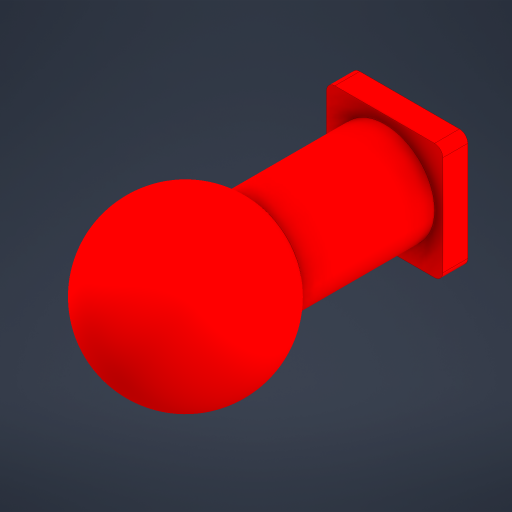
# Autodesk Inventor part: Cube Press Top
Saved by Autodesk Inventor 2023.4 (Build 274418000, 418)
## iProperties
Created: 2022-08-17
Part Number: Cube Press Top
Material: Generic
Document SubType Name: Modeling
Designer: xSibe
Density: 1 g/cm^3
Appearance: Plastic Red
Author: xSibe
Autodesk Inventor part; units mm, degrees
ref_plane "YZ Plane" through (0, 0, 0) normal (1, 0, 0) x (0, 1, 0)
ref_plane "XZ Plane" through (0, 0, 0) normal (0, 1, 0) x (-1, 0, 0)
ref_plane "XY Plane" through (0, 0, 0) normal (0, 0, 1) x (1, 0, 0)
sketch "Sketch1" plane through (0, 0, 0) normal (0, 0, 1) x (1, 0, 0)
  circle A0 centre (-21.9, -21.9) radius 1.875 projected
  circle A1 centre (21.9, 21.9) radius 1.875 projected
  circle A2 centre (21.9, -21.9) radius 1.875 projected
  circle A3 centre (-21.9, 21.9) radius 1.875 projected
  circle A4 centre (14.4, 20.8) radius 2.0734 projected
  circle A5 centre (-14.4, -20.8) radius 2.0734 projected
  circle A6 centre (14.4, -20.8) radius 2.0734 projected
  circle A7 centre (20.8, -14.4) radius 2.0734 projected
  line L0 (-17.05, 17.05) -> (-17.05, -17.05) projected
  line L1 (17.05, 17.05) -> (-17.05, 17.05) projected
  line L2 (17.05, -17.05) -> (17.05, 17.05) projected
  line L3 (-17.05, -17.05) -> (17.05, -17.05) projected
  circle A8 centre (20.8, 14.4) radius 2.0734 projected
  circle A9 centre (-14.4, 20.8) radius 2.0734 projected
  circle A10 centre (-20.8, -14.4) radius 2.0734 projected
  circle A11 centre (-20.8, 14.4) radius 2.0734 projected
  line L4 (-22.9, 24.875) -> (22.9, 24.875) projected
  arc A12 (-22.9, 24.875) -> (-24.875, 22.9) centre (-22.9, 22.9) ccw projected
  line L5 (-24.875, -22.9) -> (-24.875, 22.9) projected
  arc A13 (-24.875, -22.9) -> (-22.9, -24.875) centre (-22.9, -22.9) ccw projected
  line L6 (22.9, -24.875) -> (-22.9, -24.875) projected
  arc A14 (22.9, -24.875) -> (24.875, -22.9) centre (22.9, -22.9) ccw projected
  line L7 (24.875, 22.9) -> (24.875, -22.9) projected
  arc A15 (24.875, 22.9) -> (22.9, 24.875) centre (22.9, 22.9) ccw projected
  circle A16 centre (20.8, -14.4) radius 2.0734
  circle A17 centre (14.4, -20.8) radius 2.0734
  line L8 (-25, 25) -> (25, 25)
  line L9 (25, 25) -> (25, -25)
  line L10 (25, -25) -> (-25, -25)
  line L11 (-25, -25) -> (-25, 25)
  line L12 (-25, 25) -> (25, -25) construction
  line L13 (25, 25) -> (-25, -25) construction
  circle A18 centre (14.4, -29.2) radius 2.0734
  circle A19 centre (20.8, -35.6) radius 2.0734
  circle A20 centre (29.2, -35.6) radius 2.0734
  circle A21 centre (35.6, -29.2) radius 2.0734
  circle A22 centre (35.6, -20.8) radius 2.0734
  circle A23 centre (29.2, -14.4) radius 2.0734
  line L14 (7.5, -7.5) -> (42.5, -7.5)
  line L15 (42.5, -7.5) -> (42.5, -42.5)
  line L16 (42.5, -42.5) -> (7.5, -42.5)
  line L17 (7.5, -42.5) -> (7.5, -7.5)
  line L18 (7.5, -7.5) -> (42.5, -42.5) construction
  line L19 (42.5, -7.5) -> (7.5, -42.5) construction
  point P0 (0, 0)
  dimension "d0" = 50
  dimension "d1" = 50
  dimension "d4" = 360
  dimension "d6" = 35
  dimension "d7" = 35
  constraints: 24 end point, 8 centre point, 4 midpoint, 4 parallel, 2 coincident, 2 concentric, 2 horizontal, 2 perpendicular, 17 other
  measures "d0" distance of L9.end L10.end
  measures "d1" distance of L8.end L9.end
  measures "d6" distance of L15.end L16.end
  measures "d7" distance of L14.end L15.end
ref_plane "Work Plane1" through (-24.875, -24.875, 49.8) normal (0, 0, 1) x (1, 0, 0)
extrude "Extrusion1" add sketch "Sketch1" along normal blind 1.5 from surface at 49.8 contours A2 | L17 L14 L2 L3 | L3 L2 L14 L7 A14 L6 L17 | L6 A14 L7 L14 L9 L10 L17 | L10 L9 L14 L15 L16 L17
sketch "Sketch2" plane through (7.5, -7.5, 51.3) normal (0, 0, 1) x (1, 0, 0)
  line L0 (0, 0) -> (35, 0) projected
  line L1 (0, -35) -> (0, 0) projected
  line L2 (35, -35) -> (0, -35) projected
  line L3 (35, 0) -> (35, -35) projected
  circle A0 centre (21.7, -6.9) radius 2.0734 projected
  circle A1 centre (28.1, -21.7) radius 2.0734 projected
  circle A2 centre (13.3, -28.1) radius 2.0734 projected
  circle A3 centre (6.9, -21.7) radius 2.0734 projected
  circle A4 centre (21.7, -28.1) radius 2.0734 projected
  circle A5 centre (28.1, -13.3) radius 2.0734 projected
  circle A6 centre (13.3, -6.9) radius 2.0734 projected
  circle A7 centre (6.9, -13.3) radius 2.0734 projected
  point P0 (-7.5, 7.5)
extrude "Extrusion2" add sketch "Sketch2" along normal blind 6 contours L0 L3 L2 L1 | A0 | A1 | A2 | A3 | A4 | A5 | A6 | A7
fillet "Fillet1" radius 2.5 4 edges at (42.5, -7.5, 53.55) (7.5, -7.5, 53.55) (7.5, -42.5, 53.55) (42.5, -42.5, 53.55)
sketch "Sketch3" plane through (7.5, -7.5, 57.3) normal (0, 0, 1) x (1, 0, 0)
  arc A0 (32.5, -35) -> (35, -32.5) centre (32.5, -32.5) ccw projected
  line L0 (35, -32.5) -> (35, -2.5) projected
  arc A1 (35, -2.5) -> (32.5, 0) centre (32.5, -2.5) ccw projected
  line L1 (32.5, 0) -> (2.5, 0) projected
  arc A2 (2.5, 0) -> (0, -2.5) centre (2.5, -2.5) ccw projected
  line L2 (0, -2.5) -> (0, -32.5) projected
  arc A3 (0, -32.5) -> (2.5, -35) centre (2.5, -32.5) ccw projected
  line L3 (2.5, -35) -> (32.5, -35) projected
  line L4 (0, -17.5) -> (35, -17.5)
  circle A4 centre (17.5, -17.5) radius 15
  point P0 (-7.5, 7.5)
  dimension "d13" = 30
  constraints: 3 midpoint, 2 end point, 1 centre point
  measures "d13" diameter of A4
extrude "Extrusion3" add sketch "Sketch3" along normal blind 75 contours A4 L4 | L4 A4
fillet "Fillet2" radius 15 1 edges at (10, -25, 132.3)
ref_plane "Work Plane2" through (10, -25, 57.3) normal (0, 1, 0) x (1, 0, 0)
sketch "Sketch4" plane through (10, -25, 57.3) normal (0, 1, 0) x (1, 0, 0)
  arc A0 (0, -60) -> (30, -60) centre (15, -60) ccw projected
  circle A1 centre (15, -60) radius 25
  line L0 (15, -60) -> (15, -10)
  line L1 (15, -60) -> (15, -85)
  point P0 (-10, 57.3)
  point P1 (15, -35)
  dimension "d17" = 50
  dimension "d18" = 50
  constraints: 4 end point, 2 vertical, 1 coincident, 3 other
  measures "d18" distance of L0.start L0.end
revolve "Revolution1" add sketch "Sketch4" angle 360 about axis through (25, -25, 117.3) along (0, 0, 1) picked at (8.1418, -69.7339) contours A1 L0 L1
body "Solid1"
